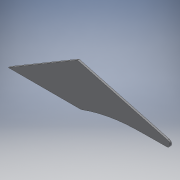
# Autodesk Inventor part: mount
Saved by Autodesk Inventor 2018.2 (Build 222227000, 227)
## iProperties
Created: 2018-03-18
Part Number: mount
Material: 一般
Document SubType Name: Modeling
Designer: ku_sk
Density: 1 g/cm^3
Appearance: 既定
Author: ku_sk
Autodesk Inventor part; units mm, degrees
ref_plane "YZ Plane" through (0, 0, 0) normal (1, 0, 0) x (0, 1, 0)
ref_plane "XZ Plane" through (0, 0, 0) normal (0, 1, 0) x (-1, 0, 0)
ref_plane "XY Plane" through (0, 0, 0) normal (0, 0, 1) x (1, 0, 0)
sketch "スケッチ1" plane through (0, 0, 0) normal (0, 1, 0) x (-1, 0, 0)
  arc A0 (-2.0246, 8.7693) -> (0, -9) centre (0, 0) ccw
  arc A1 (90, -10) -> (0, -9) centre (0, -4059.5) ccw
  arc A2 (241.9297, -38.4601) -> (90, -10) centre (79.4151, -486.2622) ccw
  arc A3 (241.9297, -38.4601) -> (245, -39) centre (245, -30) ccw
  line L0 (0, -4890.1585) -> (0, 924.451) projected
  line L1 (366.2512, 93.7925) -> (-2.0246, 8.7693)
  line L2 (541.9909, 0) -> (-101.9453, 0) projected
  line L3 (245, -39) -> (450, -39)
  line L4 (366.2512, 93.7925) -> (450, -39)
  dimension "d10" = 13
  dimension "d11" = 90
  dimension "d12" = 10
  dimension "d16" = 9
  dimension "d17" = 9
  dimension "d18" = 30
  dimension "d19" = 245
  constraints: 8 point on circle, 6 end point, 5 tangent, 4 centre point, 1 coincident, 1 horizontal, 1 point on line
  measures "d10" angle of L2 L1
  measures "d11" horizontal distance of point (0, 0) A1.start
  measures "d12" vertical distance of point (0, 0) A1.start
  measures "d16" radius of A0
  measures "d17" radius of A3
  measures "d18" distance from line of L2 A3.centre
  measures "d19" distance from line of L0 A3.centre
extrude "押し出し2" add sketch "スケッチ1" along normal mid plane 5
sketch "スケッチ2" plane through (0, 2.5, 0) normal (0, 1, 0) x (1, 0, 0)
  circle A0 centre (0, 0) radius 4 projected
  circle A1 centre (-241.7588, 15.6551) radius 4 projected
  circle A2 centre (-178.9987, -31.8162) radius 4 projected
extrude "押し出し3" cut sketch "スケッチ2" against normal through all
